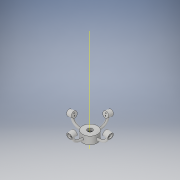
# Autodesk Inventor part: led_holder
Saved by Autodesk Inventor 2018 (Build 220112000, 112)
## iProperties
Created: 2018-06-23
Part Number: led_holder
Material: Generic
Document SubType Name: Modeling
Designer: rsmith
Density: 1 g/cm^3
Appearance: Default
Author: rsmith
Autodesk Inventor part; units mm, degrees
ref_plane "XZ Plane" through (0, 0, 0) normal (0, 1, 0) x (-1, 0, 0)
ref_plane "XY Plane" through (0, 0, 0) normal (0, 0, 1) x (1, 0, 0)
derived "led_stand.ipt"
sketch "Sketch5" plane through (0, 101.6, 0) normal (0, 1, 0) x (1, 0, 0)
  circle A0 centre (0, 0) radius 6.35
  circle A1 centre (0, 0) radius 3.175
sketch "Sketch4" plane through (0, 0, 0) normal (0, 1, 0) x (-1, 0, 0)
  circle A0 centre (0, 0) radius 6.35 projected
  circle A1 centre (0, 0) radius 3.175 projected
  circle A2 centre (0, 0) radius 9.525
  dimension "d3" = 3.175
  dimension "d4" = 3.175
  constraints: 1 centre point, 1 coincident
  measures "d3" radial gap between concentric circles of A0 A1
  measures "d4" radial gap between concentric circles of A2 A0
extrude "Extrusion1" add sketch "Sketch4" against normal blind 6.35 contours A2
extrude "Extrusion2" add sketch "Sketch4" along normal blind 3.175 contours A0 | A2
sketch "Sketch6" plane through (0, 3.175, 0) normal (0, 1, 0) x (1, 0, 0)
  circle A0 centre (0, 0) radius 9.525 projected
  line L0 (-31.75, 6.35) -> (-19.05, 6.35)
  line L1 (-19.05, 6.35) -> (-19.05, -6.35)
  line L2 (-19.05, -6.35) -> (-31.75, -6.35)
  line L3 (-31.75, -6.35) -> (-31.75, 6.35)
  circle A1 centre (0, 0) radius 9.525 projected
  line L4 (-9.525, 0) -> (-31.75, 0) construction
  dimension "d9" = 12.7
  dimension "d10" = 12.7
  dimension "d11" = 19.05
  constraints: 10 end point, 2 horizontal, 2 horizontal alignment, 2 parallel, 1 midpoint, 1 perpendicular, 1 other
  measures "d9" distance between parallel lines of L1 L3
  measures "d10" distance between parallel lines of L2 L0
  measures "d11" distance from line of point (0, 0) L1
extrude "Extrusion3" add sketch "Sketch6" along normal blind 12.7 contours L0 L1 L2 L3
sketch "Sketch7" plane through (-31.75, 3.175, 6.35) normal (0, 0, 1) x (1, 0, 0)
  line L0 (0, 0) -> (0, 12.7) projected
  line L1 (0, 10.7963) -> (10.7963, 12.7)
  line L2 (12.7, 12.7) -> (0, 12.7) projected
  line L3 (10.7963, 12.7) -> (12.7, 1.9037)
  line L4 (12.7, 1.9037) -> (1.9037, 0)
  line L5 (0, 0) -> (12.7, 0) projected
  line L6 (0, 10.7963) -> (1.9037, 0)
  line L7 (12.7, 0) -> (12.7, 12.7) projected
  point P0 (31.75, -3.175)
  dimension "d14" = 10
  constraints: 8 end point, 4 point on line, 3 perpendicular
  measures "d14" angle of L2 L1
extrude "Extrusion4" cut sketch "Sketch7" against normal through all contours L0 L6 L5 | L0 L2 L1 | L4 L7 L5 | L2 L7 L3
sketch "Sketch8" plane through (-20.9537, 15.875, 6.35) normal (0.9848078, 0.1736482, 0) x (0, 0, -1)
  line L0 (12.7, 0) -> (12.7, -10.9629) projected
  line L1 (12.7, 0) -> (0, 0) projected
  line L2 (0, -10.9629) -> (0, 0) projected
  line L3 (12.7, -10.9629) -> (0, -10.9629) projected
  circle A0 centre (6.35, -5.4814) radius 2.875
  circle A1 centre (6.35, -5.4814) radius 3.6688
  line L4 (5.85, -3.6064) -> (6.85, -3.6064)
  line L5 (6.85, -3.6064) -> (6.85, -4.6064)
  line L6 (6.85, -4.6064) -> (5.85, -4.6064)
  line L7 (5.85, -4.6064) -> (5.85, -3.6064)
  line L8 (5.85, -6.3564) -> (6.85, -6.3564)
  line L9 (6.85, -6.3564) -> (6.85, -7.3564)
  line L10 (6.85, -7.3564) -> (5.85, -7.3564)
  line L11 (5.85, -7.3564) -> (5.85, -6.3564)
  line L12 (6.35, -4.6064) -> (6.35, -6.3564) construction
  point P0 (6.35, -19.2724)
  point P1 (0, -5.4814)
  point P2 (6.35, 0)
  dimension "d17" = 1
  dimension "d18" = 1.75
  dimension "d19" = 5.75
  dimension "d20" = 0.7937
  dimension "d21" = 3.75
  constraints: 18 end point, 5 midpoint, 4 parallel, 2 centre point, 2 collinear, 2 equal length, 2 horizontal, 2 perpendicular, 1 coincident, 1 horizontal alignment, 1 vertical alignment
  measures "d17" distance between parallel lines of L6 L4
  measures "d18" distance between parallel lines of L8 L6
  measures "d19" diameter of A0
  measures "d20" radial gap between concentric circles of A1 A0
  measures "d21" distance between parallel lines of L10 L4
extrude "Extrusion5" cut sketch "Sketch8" against normal through all contours L0 L3 L2 L1 | A0 | A1 | L4 L5 L6 L7 | L8 L9 L10 L11
extrude "Extrusion6" add sketch "Sketch8" against normal blind 6.35 contours A1
extrude "Extrusion7" add sketch "Sketch8" against normal blind 4.7625 contours A0
sketch "Sketch9" plane through (0, 0, 0) normal (0, 0, 1) x (1, 0, 0)
  line L0 (-9.525, 3.175) -> (-9.525, -6.35) projected
  line L1 (9.525, 3.175) -> (-9.525, 3.175) projected
  line L2 (-19.3648, 6.8638) -> (-25.6183, 5.7612) projected
  line L3 (-20.6389, 14.0899) -> (-19.3648, 6.8638) projected
  line L4 (-22.4915, 6.3125) -> (-21.0986, -1.5875) construction
  line L5 (-21.0986, -1.5875) -> (-9.525, -1.5875) construction
  spline S0 degree 2 poles (-22.4915, 6.3125) (-21.0986, -1.5875) (-9.525, -1.5875) knots 1 1 1 2 2 2
  line L6 (-22.4915, 6.3125) -> (-22.6294, 7.0942)
  line L7 (-9.525, -1.5875) -> (-7.9375, -1.5875)
  point P0 (0, 0)
  dimension "d28" = 0.7937
  dimension "d29" = 1.5875
  constraints: 4 end point, 2 midpoint, 2 parallel, 1 collinear, 1 point on line, 3 other
  measures "d28" distance from line of L2 L6.end
  measures "d29" distance of L7.end L5.end
ref_plane "Work Plane1" through (-9.525, 0, 0) normal (1, 0, 0) x (0, 1, 0)
sketch "Sketch10" plane through (-9.525, 0, 0) normal (1, 0, 0) x (0, 1, 0)
  circle A0 centre (-1.5875, 0) radius 1.5875
  point P0 (0, 0)
  dimension "d30" = 3.175
  constraints: 1 centre point, 1 coincident
  measures "d30" diameter of A0
sweep "Sweep1" add profiles "Sketch10" path "Sketch9" path curves L7 S0 L6
pattern_circular "Circular Pattern1" count 4 over 360 about axis through (0, -10, 0) along (0, 1, 0) of "Sweep1", "Extrusion6", "Extrusion7"
equation "\"d4\" = d3"
body "Solid2"
